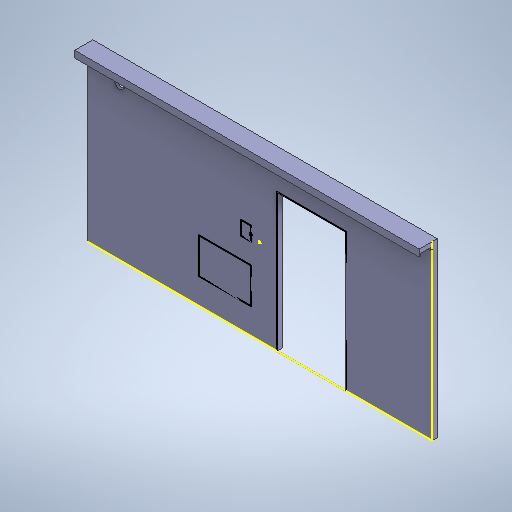
# Autodesk Inventor part: FrontWall
Saved by Autodesk Inventor 2026.2 (Build 302298010, 298A)
## iProperties
Created: 2026-03-19
Part Number: FrontWall
Material: Ogólny
Document SubType Name: Modeling
Designer: Patryk
Density: 1 g/cm^3
Appearance: Domyślna
Author: Patryk
Autodesk Inventor part; units mm, degrees
ref_plane "YZ Plane" through (0, 0, 0) normal (1, 0, 0) x (0, 1, 0)
ref_plane "XZ Plane" through (0, 0, 0) normal (0, 1, 0) x (-1, 0, 0)
ref_plane "XY Plane" through (0, 0, 0) normal (0, 0, 1) x (1, 0, 0)
sketch "Szkic1" plane through (0, 0, 0) normal (0, 0, 1) x (1, 0, 0)
  line L0 (200, -100) -> (-200, -100)
  line L1 (-200, -100) -> (-200, 100)
  line L2 (-200, 100) -> (200, 100)
  line L3 (200, 100) -> (200, -100)
  line L4 (200, -100) -> (-200, 100) construction
  line L5 (-200, -100) -> (200, 100) construction
  point P0 (0, 0)
  dimension "d0" = 400
  dimension "d1" = 200
  constraints: 12 end point, 2 midpoint, 2 parallel, 1 horizontal, 1 perpendicular
  measures "d0" distance of L1.end L2.end
  measures "d1" distance of L0.end L1.end
extrude "Wyciągnięcie proste1" add sketch "Szkic1" along normal mid plane 6
sketch "Szkic2" plane through (0, 0, 3) normal (0, 0, 1) x (1, 0, 0)
  line L0 (-200, -100) -> (200, -100) projected
  line L1 (20, -100) -> (100, -100)
  line L2 (100, -100) -> (100, 60)
  line L3 (100, 60) -> (20, 60)
  line L4 (20, 60) -> (20, -100)
  line L5 (200, -100) -> (200, 100) projected
  line L6 (-22, 11) -> (-10, 11)
  line L7 (-10, 11) -> (-10, -5)
  line L8 (-10, -5) -> (-22, -5)
  line L9 (-22, -5) -> (-22, 11)
  line L10 (-71, -29) -> (-10, -29)
  line L11 (-10, -29) -> (-10, -70)
  line L12 (-10, -70) -> (-71, -70)
  line L13 (-71, -70) -> (-71, -29)
  point P0 (0, 0)
  point P1 (-10, 3)
  dimension "d4" = 80
  dimension "d5" = 160
  dimension "d6" = 100
  dimension "d7" = 16
  dimension "d8" = 12
  dimension "d9" = 95
  dimension "d10" = 61
  dimension "d11" = 41
  dimension "d12" = 30
  dimension "d13" = 30
  dimension "d14" = 30
  constraints: 24 end point, 6 parallel, 3 horizontal, 3 perpendicular, 1 midpoint, 1 point on line
  measures "d4" distance of L3.end L2.end
  measures "d5" distance of L2.end L1.end
  measures "d6" distance between parallel lines of L5 L2
  measures "d7" distance of L8.end L6.start
  measures "d8" distance of L6.start L6.end
  measures "d9" distance between parallel lines of L0 L8
  measures "d10" distance of L10.start L10.end
  measures "d11" distance of L12.end L10.start
  measures "d12" distance between parallel lines of L0 L12
  measures "d13" distance between parallel lines of L4 L11
  measures "d14" distance from line of L4 point (-10, 3)
extrude "Wyciągnięcie proste2" cut sketch "Szkic2" against normal through all contours L4 L3 L2 L0
sketch "Szkic3" plane through (0, 0, -3) normal (0, 0, -1) x (-1, 0, 0)
  line L0 (71, -29) -> (10, -29) projected
  line L1 (71, -70) -> (71, -29) projected
  line L2 (10, -70) -> (71, -70) projected
  line L3 (10, -29) -> (10, -70) projected
  line L4 (10, -5) -> (22, -5) projected
  line L5 (22, -5) -> (22, 11) projected
  line L6 (22, 11) -> (10, 11) projected
  line L7 (10, 11) -> (10, -5) projected
  point P0 (0, 0)
  point P1 (10, 3)
extrude "Wyciągnięcie proste3" cut sketch "Szkic3" against normal blind 5 contours L7 L6 L5 L4
sketch "Szkic4" plane through (0, 0, -3) normal (0, 0, -1) x (-1, 0, 0)
  line L0 (71, -29) -> (10, -29) projected
  line L1 (71, -70) -> (71, -29) projected
  line L2 (10, -70) -> (71, -70) projected
  line L3 (10, -29) -> (10, -70) projected
  point P0 (0, 0)
extrude "Wyciągnięcie proste4" cut sketch "Szkic4" against normal blind 3
sketch "Szkic6" plane through (0, 0, -3) normal (0, 0, -1) x (-1, 0, 0)
  line L0 (22, -5) -> (10, -5) projected
  line L1 (12, -5) -> (12, -21)
  line L2 (12, -21) -> (82, -21)
  line L3 (82, -21) -> (82, -40)
  line L4 (82, -40) -> (71, -40)
  line L5 (71, -29) -> (71, -70) projected
  line L6 (71, -60) -> (82, -60)
  line L7 (71, -70) -> (10, -70) projected
  line L8 (10, -70) -> (10, -29) projected
  line L9 (10, -29) -> (71, -29) projected
  line L10 (71, -29) -> (71, -70) projected
  line L11 (10, 11) -> (22, 11) projected
  line L12 (22, 11) -> (22, -5) projected
  line L13 (22, -5) -> (10, -5) projected
  line L14 (10, -5) -> (10, 11) projected
  line L15 (-20, 60) -> (-20, -100) projected
  line L16 (-20, -100) -> (200, -100) projected
  line L17 (200, -100) -> (200, 100) projected
  line L18 (200, 100) -> (-200, 100) projected
  line L19 (-200, 100) -> (-200, -100) projected
  line L20 (-200, -100) -> (-100, -100) projected
  line L21 (-100, -100) -> (-100, 60) projected
  line L22 (-100, 60) -> (-20, 60) projected
  line L23 (82, -60) -> (82, -100)
  line L24 (-20, -100) -> (200, -100) projected
  line L25 (20, -5) -> (20, -13)
  line L26 (20, -13) -> (90, -13)
  line L27 (90, -13) -> (90, -100)
  point P0 (0, 0)
  point P1 (12, -13)
  dimension "d21" = 8
  dimension "d22" = 32
  dimension "d23" = 8
  dimension "d24" = 8
  dimension "d25" = 20
  dimension "d26" = 40
  dimension "d27" = 8
  dimension "d28" = 8
  constraints: 18 end point, 4 perpendicular, 4 point on line, 2 horizontal, 2 midpoint, 2 vertical
  measures "d21" distance between parallel lines of L25 L1
  measures "d22" distance from line of L15 point (12, -13)
  measures "d23" distance between parallel lines of L2 L26
  measures "d24" distance between parallel lines of L2 L9
  measures "d25" distance between parallel lines of L6 L4
  measures "d26" distance between parallel lines of L16 L6
  measures "d27" distance between parallel lines of L27 L3
  measures "d28" distance between parallel lines of L27 L23
extrude "Wyciągnięcie proste5" cut sketch "Szkic6" against normal blind 3 contours L25 L26 L27 L16 L23 L6 L5 L4 L3 L2 L1 L0
sketch "Szkic7" plane through (0, 0, 3) normal (0, 0, 1) x (1, 0, 0)
  line L0 (-200, 100) -> (200, 100) projected
  line L1 (200, 100) -> (200, -100) projected
  line L2 (-200, 100) -> (200, 100)
  line L3 (200, 100) -> (200, 92)
  line L4 (200, 92) -> (-200, 92)
  line L5 (-200, 92) -> (-200, 100)
  point P0 (0, 0)
  dimension "d31" = 8
  constraints: 8 end point, 2 parallel, 1 horizontal, 1 perpendicular, 1 point on line
  measures "d31" distance between parallel lines of L4 L0
extrude "Wyciągnięcie proste6" add sketch "Szkic7" along normal blind 15
sketch "Szkic8" plane through (-200, 92, 3) normal (0, -1, 0) x (1, 0, 0)
  line L0 (400, 15) -> (400, -6) projected
  line L1 (0, -6) -> (0, 15) projected
  line L2 (400, 13) -> (0, 13)
  line L3 (0, 13) -> (0, 2)
  line L4 (0, 2) -> (400, 2)
  line L5 (400, 2) -> (400, 13)
  line L6 (0, 15) -> (400, 15) projected
  point P0 (200, -3)
  point P1 (0, 13)
  dimension "d34" = 11
  dimension "d35" = 2
  constraints: 8 end point, 2 parallel, 2 point on line, 1 horizontal, 1 perpendicular
  measures "d34" distance between parallel lines of L4 L2
  measures "d35" distance between parallel lines of L2 L6
extrude "Wyciągnięcie proste7" cut sketch "Szkic8" against normal blind 3 contours L0 L4 L1 L2
sketch "Szkic9" plane through (0, 0, -3) normal (0, 0, -1) x (-1, 0, 0)
  line L0 (156, 85) -> (170, 85)
  line L1 (170, 85) -> (170, 55)
  line L2 (170, 55) -> (156, 55)
  line L3 (156, 55) -> (156, 85)
  line L4 (200, -100) -> (200, 100) projected
  line L5 (200, 100) -> (-200, 100) projected
  circle A0 centre (163, 78) radius 6
  line L6 (90, -100) -> (200, -100) projected
  line L7 (159, 55) -> (159, -100)
  line L8 (167, 55) -> (167, -100)
  point P0 (0, 0)
  point P1 (163, 55)
  dimension "d38" = 14
  dimension "d39" = 30
  dimension "d40" = 30
  dimension "d41" = 15
  dimension "d42" = 12
  dimension "d43" = 23
  dimension "d44" = 7
  dimension "d49" = 8
  dimension "d50" = 33
  constraints: 12 end point, 4 point on line, 3 perpendicular, 2 parallel, 1 centre point, 1 horizontal, 1 midpoint
  measures "d38" distance of L1.end L2.end
  measures "d39" distance of L0.end L1.end
  measures "d40" distance between parallel lines of L4 L1
  measures "d41" distance between parallel lines of L5 L0
  measures "d42" diameter of A0
  measures "d43" distance of point (163, 55) A0.centre
  measures "d44" distance from line of L1 A0.centre
  measures "d49" distance between parallel lines of L8 L7
  measures "d50" distance between parallel lines of L4 L8
extrude "Wyciągnięcie proste8" cut sketch "Szkic9" against normal blind 6 contours A0
extrude "Wyciągnięcie proste9" cut sketch "Szkic9" against normal blind 3 contours L0 L1 L2 L3
extrude "Wyciągnięcie proste10" cut sketch "Szkic9" against normal blind 3 contours L2 L8 L6 L7
